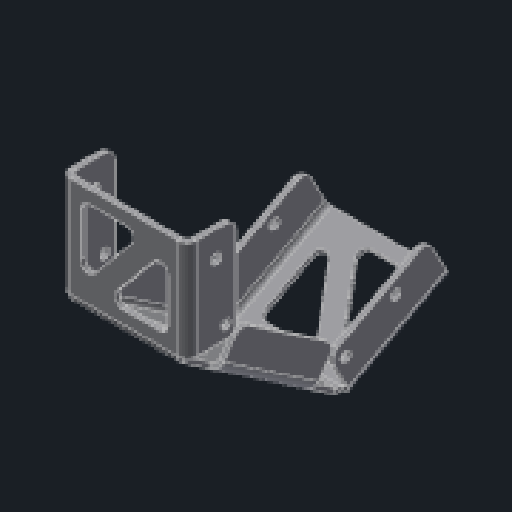
# Autodesk Inventor part: HipCoverTop
Saved by Autodesk Inventor 2025.2 (Build 292293000, 293)
## iProperties
Created: 2020-05-24
Part Number: HipCoverTop
Material: Generic
Document SubType Name: Sheet Metal
Designer: valer
Density: 1 g/cm^3
Sheet Metal Rule: Default
Appearance: Default
Author: valer
Autodesk Inventor part; units mm, degrees
ref_plane "YZ Plane" through (0, 0, 0) normal (1, 0, 0) x (0, 1, 0)
ref_plane "XZ Plane" through (0, 0, 0) normal (0, 1, 0) x (-1, 0, 0)
ref_plane "XY Plane" through (0, 0, 0) normal (0, 0, 1) x (1, 0, 0)
sketch "Base" plane through (0, 0, 0) normal (0, 0, 1) x (1, 0, 0)
  line L0 (0, 0) -> (41, 0)
  line L1 (41, 0) -> (41, -65.2018)
  line L2 (41, -65.2018) -> (0, -65.2018)
  line L3 (0, -65.2018) -> (0, 0)
  dimension "d0" = 65.2018
  dimension "d1" = 41
  measures "d0" distance of L2.end L0.start
  measures "d1" distance of L0.start L0.end
extrude "Plate1" add sketch "Base" along normal blind 3.048
sketch "Sketch2" plane through (3.048, 0, 3.048) normal (-1, 0, 0) x (0, -1, 0)
  line L0 (65.2018, 0) -> (0, 0)
  line L1 (0, 0) -> (0, -31.75)
  line L2 (0, -31.75) -> (65.2018, -31.75)
  line L3 (65.2018, -31.75) -> (65.2018, 0)
  constraints: 6 end point, 1 horizontal, 1 perpendicular, 1 vertical
edge flange "MountFeature" height 31.75 angle 90 thickness 3.048 bend radius 3.048 thickness toward (-1, 0, 0) relief straight relief width 3.048 relief depth 1.524 edges at (0, -32.6009, 0) wall of the first edge with corners at (3.048, -65.2018, 3.048) (3.048, 0, 3.048) (3.048, 0, -28.702) (3.048, -65.2018, -28.702)
bend "Bend1"
corner "Corner1"
sketch "MountHoles" plane through (0, -65.2018, -28.702) normal (-1, 0, 0) x (0, 0, 1)
  arc A0 (10.150845, 50.036867) -> (15.493805, 46.605354) centre (12.822325, 48.32111) ccw
  arc A1 (7.802732, 11.528906) -> (5.106142, 5.779914) centre (6.454437, 8.65441) ccw
hole "MountHolesFeature" at (0, -16.88069, -15.879675) at (0, -56.54739, -22.247563) direction (1, 0, 0) diameter 6.35 end through all
mirror "MirrorFeature" about plane through (41, 0, 0) normal (1, 0, 0)
sketch "GenerativeCut1" plane through (0, 0, 3.048) normal (0, 0, 1) x (1, 0, 0)
  line L0 (12.7, -8.466667) -> (12.7, -56.735133)
  line L1 (12.7, -56.735133) -> (52.790691, -8.466667)
  line L2 (52.790691, -8.466667) -> (12.7, -8.466667)
  line L3 (75.904, 0) -> (6.096, 0)
  line L4 (29.209309, -56.735133) -> (69.3, -8.466667)
  line L5 (69.3, -8.466667) -> (69.3, -56.735133)
  line L6 (69.3, -56.735133) -> (29.209309, -56.735133)
  line L7 (52.790691, -8.466667) -> (69.3, -8.466667) construction
  line L8 (12.7, -56.735133) -> (29.209309, -56.735133) construction
  line L9 (0, -65.2018) -> (0, 0)
  line L10 (82, -65.2018) -> (82, 0)
  line L11 (75.904, -65.2018) -> (6.096, -65.2018)
  dimension "d23" = 8.46667
  dimension "d24" = 12.7
  dimension "d25" = 12.7
  dimension "d26" = 8.46667
  dimension "d27" = 12.7
  constraints: 16 end point, 2 parallel, 2 perpendicular, 1 collinear, 1 horizontal, 1 vertical
  measures "d23" distance between parallel lines of L3 L2
  measures "d24" distance between parallel lines of L9 L0
  measures "d25" distance between parallel lines of L5 L10
  measures "d26" distance between parallel lines of L11 L6
  measures "d27" distance between parallel lines of L4 L1
extrude "GenerativeCut1Feature" cut sketch "GenerativeCut1" against normal blind 25.4
fillet "GenerativeCut1FilletsFeature" radius 5.08 6 edges at (12.7, -8.4667, 1.524) (12.7, -56.7351, 1.524) (52.7907, -8.4667, 1.524) (69.3, -8.4667, 1.524) (29.2093, -56.7351, 1.524) (69.3, -56.7351, 1.524)
sketch "Sketch5" plane through (75.904, -67.724236, -1.33697) normal (0, -0.8275708, 0.5613614) x (1, 0, 0)
  line L0 (-69.808, 0) -> (0, 0)
  line L1 (0, 0) -> (0, 118.688928)
  line L2 (0, 118.688928) -> (-69.808, 118.688928)
  line L3 (-69.808, 118.688928) -> (-69.808, 0)
  constraints: 6 end point, 1 horizontal, 1 perpendicular, 1 vertical
edge flange "KneeFlangeFeature" height 121.92 angle 55.85 thickness 3.048 bend radius 3.048 thickness toward (0, -0.8275708, 0.5613614) relief straight relief width 3.048 relief depth 1.524 edges at (41, -65.2018, 3.048) wall of the first edge with corners at (6.096, -67.724236, -1.33697) (75.904, -67.724236, -1.33697) (75.904, -134.351618, -99.560458) (6.096, -134.351618, -99.560458)
bend "Bend2"
corner "Corner2"
sketch "Sketch6" plane through (6.096, -134.519407, -102.704315) normal (0, -0.8826196, -0.4700879) x (1, 0, 0)
  line L0 (69.808, 0) -> (0, 0)
  line L1 (0, 0) -> (0, -72.523383)
  line L2 (0, -72.523383) -> (69.808, -72.523383)
  line L3 (69.808, -72.523383) -> (69.808, 0)
  constraints: 8 end point
edge flange "KneeBottomFlangeFeature" height 76.2 angle 62.19 thickness 3.048 bend radius 3.048 thickness toward (0, -0.8826196, -0.4700879) relief straight relief width 3.048 relief depth 1.524 edges at (41, -134.351618, -99.560458) wall of the first edge with corners at (75.904, -134.519407, -102.704315) (6.096, -134.519407, -102.704315) (6.096, -100.427045, -166.714876) (75.904, -100.427045, -166.714876)
bend "Bend3"
corner "Corner3"
sketch "Sketch8" plane through (3.048, -131.829183, -101.271487) normal (-1, 0, 0) x (0, -1, 0)
  line L0 (-34.092362, -64.010561) -> (0, 0)
  line L1 (0, 0) -> (-22.642724, 12.059634)
  line L2 (-22.642724, 12.059634) -> (-56.735086, -51.950927)
  line L3 (-56.735086, -51.950927) -> (-34.092362, -64.010561)
  constraints: 6 end point, 1 perpendicular, 2 other
edge flange "KneeBottomSidesFeature" height 31.75 angle 90 thickness 3.048 bend radius 3.048 thickness toward (-1, 0, 0) relief straight relief width 3.048 relief depth 1.524 corner gap 3.048 corner form 0 edges at (6.096, -117.473226, -134.709596) (75.904, -117.473226, -134.709596) wall of the first edge with corners at (3.048, -97.736821, -165.282049) (3.048, -131.829183, -101.271487) (3.048, -109.186459, -89.211853) (3.048, -75.094097, -153.222415)
bend "Bend4"
corner "Corner4"
fillet "OutsideFilletsFeature" radius 6.35 8 edges at (1.524, -65.2018, -28.702) (1.524, 0, -28.702) (1.524, -109.1865, -89.2119) (80.476, -75.0941, -153.2224) (1.524, -75.0941, -153.2224) (80.476, -109.1865, -89.2119) (80.476, -65.2018, -28.702) (80.476, 0, -28.702)
sketch "Sketch10" plane through (6.096, -70.246671, 0.374059) normal (0, -0.8275708, 0.5613614) x (1, 0, 0)
  line L0 (-3.048, -18.760781) -> (-6.096, -18.760781)
  line L1 (-3.048, -98.227084) -> (-6.096, -98.227084)
  line L2 (-6.096, -21.300781) -> (0, -21.300781)
  line L3 (0, -21.300781) -> (0, -95.687084)
  line L4 (0, -95.687084) -> (-6.096, -95.687084)
  line L5 (-6.096, -95.687084) -> (-6.096, -21.300781)
  line L6 (-6.096, 0) -> (-6.096, -15.975426)
  line L7 (0, 0) -> (0, -118.688928)
  point P0 (-6.096, 39.124209)
  dimension "d65" = 2.54
  dimension "d66" = 2.54
  constraints: 8 end point, 2 collinear, 2 parallel, 1 horizontal, 1 perpendicular
  measures "d65" distance between parallel lines of L0 L2
  measures "d66" distance between parallel lines of L1 L4
sheet face with bend "SideFlangeBaseFeature" sketch "Sketch10" thickness 3.048 toward (0, 0.8275708, -0.5613614) bend radius 3.048 relief straight relief width 3.048 relief depth 1.524
bend "Bend5"
sketch "Sketch11" plane through (3.048, -82.204108, -17.253845) normal (-1, 0, 0) x (0, -1, 0)
  line L0 (41.757599, -61.55993) -> (0, 0)
  line L1 (0, 0) -> (-21.020298, -14.25858)
  line L2 (-21.020298, -14.25858) -> (20.737301, -75.818509)
  line L3 (20.737301, -75.818509) -> (41.757599, -61.55993)
  constraints: 6 end point, 1 perpendicular, 2 other
edge flange "SideFlangeFeature" height 25.4 angle 90 thickness 3.048 bend radius 3.048 thickness toward (-1, 0, 0) relief straight relief width 3.048 relief depth 1.524 edges at (0, -100.560472, -49.744839) wall of the first edge with corners at (3.048, -123.961707, -78.813774) (3.048, -82.204108, -17.253845) (3.048, -61.18381, -31.512424) (3.048, -102.941409, -93.072354)
bend "Bend6"
corner "Corner5"
ref_plane "MiddlePlane" through (41, -97.736821, -165.282049) normal (-1, 0, 0) x (0, -0.4700879, 0.8826196)
mirror "SideFlangeMirrorFeature" about plane through (41, -97.736821, -165.282049) normal (-1, 0, 0) of "SideFlangeFeature"
fillet "SideFlangeFilletsFeature" radius 6.35 4 edges at (1.524, -102.9414, -93.0724) (80.476, -102.9414, -93.0724) (1.524, -61.1838, -31.5124) (80.476, -61.1838, -31.5124)
sketch "KneeMountHoles" plane through (0, -97.736821, -165.282049) normal (-1, 0, 0) x (0, -0.4700879, 0.8826196)
  arc A0 (30.823709, 17.304472) -> (24.557799, 18.334458) centre (27.690754, 17.819465) ccw
  arc A1 (68.203567, 17.535556) -> (62.188704, 15.499893) centre (65.196135, 16.517724) ccw
  point P0 (99.936287, 163.961521)
hole "KneeMountHolesFeature" at (0, -113.805865, -99.973878) at (0, -95.026098, -132.464931) direction (1, 0, 0) diameter 6.35 end through all
sketch "Rais" plane through (6.096, -70.246671, 0.374059) normal (0, -0.8275708, 0.5613614) x (1, 0, 0)
  line L0 (69.808, 0) -> (0, 0) construction
  line L1 (0, -118.688928) -> (69.808, -118.688928) construction
  line L2 (0, 0) -> (69.808, 0) construction
  line L3 (34.904, 0) -> (34.904, -118.688928) construction
  line L4 (0, -118.688928) -> (69.808, -118.688928) construction
  line L5 (26.694128, -42.590128) -> (17.713872, -33.609872) construction
  line L6 (24.449064, -44.835192) -> (15.468808, -35.854936)
  line L7 (19.958936, -31.364808) -> (28.939192, -40.345064)
  arc A0 (24.449064, -44.835192) -> (28.939192, -40.345064) centre (26.694128, -42.590128) ccw
  arc A1 (19.958936, -31.364808) -> (15.468808, -35.854936) centre (17.713872, -33.609872) ccw
  line L8 (0, -21.300781) -> (0, -95.687084) construction
  line L9 (0, -58.493932) -> (69.808, -58.493932) construction
  line L10 (69.808, -95.687084) -> (69.808, -21.300781) construction
  line L11 (45.358936, -44.835192) -> (54.339192, -35.854936)
  line L12 (49.849064, -31.364808) -> (40.868808, -40.345064)
  arc A2 (40.868808, -40.345064) -> (45.358936, -44.835192) centre (43.113872, -42.590128) ccw
  arc A3 (54.339192, -35.854936) -> (49.849064, -31.364808) centre (52.094128, -33.609872) ccw
  line L13 (24.449064, -72.152673) -> (15.468808, -81.132929)
  line L14 (19.958936, -85.623057) -> (28.939192, -76.642801)
  arc A4 (28.939192, -76.642801) -> (24.449064, -72.152673) centre (26.694128, -74.397737) ccw
  arc A5 (15.468808, -81.132929) -> (19.958936, -85.623057) centre (17.713872, -83.377993) ccw
  line L15 (45.358936, -72.152673) -> (54.339192, -81.132929)
  arc A6 (49.849064, -85.623057) -> (54.339192, -81.132929) centre (52.094128, -83.377993) ccw
  line L16 (49.849064, -85.623057) -> (40.868808, -76.642801)
  arc A7 (45.358936, -72.152673) -> (40.868808, -76.642801) centre (43.113872, -74.397737) ccw
  point P0 (-6.096, 39.124209)
  point P1 (22.204, -38.1)
  dimension "d101" = 3.175
  dimension "d102" = 12.7
  dimension "d103" = 12.7
  dimension "d104" = 38.1
  dimension "d105" = 45
  constraints: 24 end point, 18 symmetric about line, 16 point on circle, 8 centre point, 5 midpoint, 4 tangent, 1 parallel, 6 other
  measures "d101" radius of A1
  measures "d102" distance from line of L3 point (22.204, -38.1)
  measures "d103" distance of L5.start L5.end
  measures "d104" distance from line of L0 point (22.204, -38.1)
  measures "d105" angle of L3 L5
extrude "RailsFeature" cut sketch "Rais" against normal blind 25.4
sketch "GenerativeCut2" plane through (6.096, -137.209632, -104.137143) normal (0, -0.8826196, -0.4700879) x (1, 0, 0)
  line L0 (8.466667, -8.466667) -> (8.466667, -64.056717)
  line L1 (8.466667, -64.056717) -> (46.015595, -8.466667)
  line L2 (46.015595, -8.466667) -> (8.466667, -8.466667)
  line L3 (23.792405, -64.056717) -> (61.341333, -8.466667)
  line L4 (61.341333, -8.466667) -> (61.341333, -64.056717)
  line L5 (61.341333, -64.056717) -> (23.792405, -64.056717)
  line L6 (46.015595, -8.466667) -> (61.341333, -8.466667) construction
  line L7 (8.466667, -64.056717) -> (23.792405, -64.056717) construction
  line L8 (69.808, 0) -> (0, 0)
  line L9 (0, -72.523383) -> (0, 0)
  line L10 (69.808, -72.523383) -> (0, -72.523383)
  line L11 (69.808, 0) -> (69.808, -72.523383)
  point P0 (-6.096, 27.412903)
  dimension "d124" = 12.7
  dimension "d125" = 8.46667
  dimension "d126" = 8.46667
  dimension "d127" = 8.46667
  dimension "d128" = 8.46667
  constraints: 16 end point, 2 perpendicular, 1 collinear, 1 horizontal, 1 parallel, 1 vertical
  measures "d124" distance between parallel lines of L3 L1
  measures "d125" distance between parallel lines of L8 L2
  measures "d126" distance between parallel lines of L9 L0
  measures "d127" distance between parallel lines of L11 L4
  measures "d128" distance between parallel lines of L10 L5
extrude "GenerativeCut2Feature" cut sketch "GenerativeCut2" against normal blind 25.4 contours L2 L1 L0 | L3 L4 L5
fillet "GenerativeCut2FilletsFeature" radius 5.08 6 edges at (14.5627, -131.8844, -110.8936) (52.1116, -131.8844, -110.8936) (14.5627, -105.7522, -159.9584) (29.8884, -105.7522, -159.9584) (67.4373, -131.8844, -110.8936) (67.4373, -105.7522, -159.9584)
equation "\"d20\" = Thickness"
equation "\"d25\" = d24"
equation "\"d26\" = d23"
equation "\"d27\" = d24"
equation "\"d88\" = Thickness"
equation "\"d124\" = d121"
equation "\"d2\" = Thickness"
equation "\"d3\" = BendReliefWidth"
equation "\"d4\" = BendReliefDepth"
equation "\"d5\" = MinimumRemnant"
equation "\"d6\" = TransitionRadius"
equation "\"d9\" = BendRadius"
equation "\"d10\" = CornerReliefSize"
equation "\"d11\" = GapSize"
equation "\"d12\" = JacobiRadiusSize"
equation "\"d31\" = BendReliefWidth"
equation "\"d32\" = BendReliefDepth"
equation "\"d33\" = MinimumRemnant"
equation "\"d34\" = TransitionRadius"
equation "\"d37\" = BendRadius"
equation "\"d38\" = CornerReliefSize"
equation "\"d39\" = GapSize"
equation "\"d40\" = JacobiRadiusSize"
equation "\"d41\" = BendReliefWidth"
equation "\"d42\" = BendReliefDepth"
equation "\"d43\" = MinimumRemnant"
equation "\"d44\" = TransitionRadius"
equation "\"d47\" = BendRadius"
equation "\"d48\" = CornerReliefSize"
equation "\"d49\" = GapSize"
equation "\"d50\" = JacobiRadiusSize"
equation "\"d51\" = BendReliefWidth"
equation "\"d52\" = BendReliefDepth"
equation "\"d53\" = MinimumRemnant"
equation "\"d54\" = TransitionRadius"
equation "\"d57\" = BendRadius"
equation "\"d58\" = CornerReliefSize"
equation "\"d59\" = GapSize"
equation "\"d60\" = JacobiRadiusSize"
equation "\"d66\" = d65"
equation "\"d67\" = BendRadius"
equation "\"d68\" = BendReliefWidth"
equation "\"d70\" = MinimumRemnant"
equation "\"d69\" = BendReliefDepth"
equation "\"d71\" = TransitionRadius"
equation "\"d72\" = BendReliefWidth"
equation "\"d73\" = BendReliefDepth"
equation "\"d74\" = MinimumRemnant"
equation "\"d75\" = TransitionRadius"
equation "\"d78\" = BendRadius"
equation "\"d79\" = CornerReliefSize"
equation "\"d80\" = GapSize"
equation "\"d81\" = JacobiRadiusSize"
equation "\"BendRadius\" = Thickness"
equation "\"BendReliefWidth\" = Thickness"
equation "\"BendReliefDepth\" = 0.5 * Thickness"
equation "\"CornerReliefSize\" = 4 * Thickness"
equation "\"MinimumRemnant\" = 2 * Thickness"
equation "\"TransitionRadius\" = BendRadius"
equation "\"JacobiRadiusSize\" = BendRadius"
equation "\"GapSize\" = Thickness"
equation "\"Thickness\" = 3.048"
equation "\"d121\" = 12.7"
body "Solid1"
